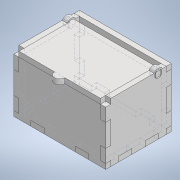
# Autodesk Inventor part: music box
Saved by Autodesk Inventor 2020 (Build 240168000, 168)
## iProperties
Created: 2021-07-07
Part Number: music box
Material: Generic
Document SubType Name: Modeling
Designer: Administrator
Density: 1 g/cm^3
Appearance: Default
Author: Administrator
Autodesk Inventor part; units mm, degrees
ref_plane "YZ Plane" through (0, 0, 0) normal (1, 0, 0) x (0, 1, 0)
ref_plane "XZ Plane" through (0, 0, 0) normal (0, 1, 0) x (-1, 0, 0)
ref_plane "XY Plane" through (0, 0, 0) normal (0, 0, 1) x (1, 0, 0)
sketch "Sketch1" plane through (0, 0, 0) normal (0, 0, 1) x (1, 0, 0)
  line L0 (-35, -22.5) -> (35, -22.5)
  line L1 (35, -22.5) -> (35, 22.5)
  line L2 (35, 22.5) -> (-35, 22.5)
  line L3 (-35, 22.5) -> (-35, -22.5)
  line L4 (-35, -22.5) -> (35, 22.5) construction
  line L5 (35, -22.5) -> (-35, 22.5) construction
  line L6 (-35, 0) -> (35, 0) construction
  line L7 (0, 22.5) -> (0, -22.5) construction
  line L8 (-35, 18.6) -> (-31.1, 18.6)
  line L9 (-31.1, 18.6) -> (-31.1, 8.6)
  line L10 (-31.1, 8.6) -> (-35, 8.6)
  line L11 (-35, 8.6) -> (-35, 18.6)
  line L12 (-35, -18.6) -> (-31.1, -18.6)
  line L13 (-31.1, -18.6) -> (-31.1, -8.6)
  line L14 (-31.1, -8.6) -> (-35, -8.6)
  line L15 (35, 18.6) -> (31.1, 18.6)
  line L16 (31.1, 18.6) -> (31.1, 8.6)
  line L17 (31.1, 8.6) -> (35, 8.6)
  line L18 (31.1, -18.6) -> (31.1, -8.6)
  line L19 (31.1, -8.6) -> (35, -8.6)
  line L20 (35, -18.6) -> (31.1, -18.6)
  line L21 (-22, -22.5) -> (-12, -22.5)
  line L22 (-12, -22.5) -> (-12, -18.6)
  line L23 (-12, -18.6) -> (-22, -18.6)
  line L24 (-22, -18.6) -> (-22, -22.5)
  line L25 (12, -22.5) -> (12, -18.6)
  line L26 (12, -18.6) -> (22, -18.6)
  line L27 (22, -18.6) -> (22, -22.5)
  point P0 (0, 0)
  point P1 (-35, -18.6)
  point P2 (35, -18.6)
  point P3 (35, -8.6)
  point P4 (35, 8.6)
  point P5 (35, 18.6)
  point P6 (-35, 8.6)
  point P7 (-35, -8.6)
  dimension "d0" = 70
  dimension "d1" = 45
  dimension "d2" = 3.9
  dimension "d3" = 10
  dimension "d4" = 3.9
  dimension "d7" = 10
  dimension "d8" = 3.9
  dimension "d9" = 12
  constraints: 56 end point, 16 symmetric about line, 6 midpoint, 6 parallel, 3 horizontal, 3 perpendicular, 2 point on line
  measures "d0" distance of L2.end L1.end
  measures "d1" distance of L1.end L0.end
  measures "d2" distance of L9.end L10.end
  measures "d3" distance of L8.end L9.end
  measures "d4" distance between parallel lines of L2 L8
  measures "d7" distance of L23.end L22.end
  measures "d8" distance of L22.end L21.end
  measures "d9" distance between parallel lines of L7 L22
extrude "Extrusion1" add sketch "Sketch1" along normal blind 3.9 contours L3 L12 L13 L14 L10 L9 L8 L2 L1 L15 L16 L17 L19 L18 L20 L0 L27 L26 L25 L22 L23 L24
sketch "Sketch2" plane through (-35, -8.6, 0) normal (-1, 0, 0) x (0, 0, 1)
  line L0 (50, -13.9) -> (0, -13.9)
  line L1 (0, -13.9) -> (0, 31.1)
  line L2 (0, 31.1) -> (50, 31.1)
  line L3 (50, 31.1) -> (50, -13.9)
  line L4 (50, -13.9) -> (0, 31.1) construction
  line L5 (0, -13.9) -> (50, 31.1) construction
  line L6 (3.9, 31.1) -> (3.9, 27.2) projected
  line L7 (0, 31.1) -> (0, 27.2) projected
  line L8 (3.9, 27.2) -> (0, 27.2)
  line L9 (0, 27.2) -> (0, 31.1)
  line L10 (0, 31.1) -> (3.9, 31.1)
  line L11 (3.9, 31.1) -> (3.9, 27.2)
  line L12 (25, 31.1) -> (25, -13.9) construction
  line L13 (0, 8.6) -> (50, 8.6) construction
  line L14 (0, 0) -> (0, -10) projected
  line L15 (0, -10) -> (3.9, -10)
  line L16 (3.9, -10) -> (3.9, -13.9)
  line L17 (3.9, -13.9) -> (0, -13.9)
  line L18 (0, -13.9) -> (0, -10)
  line L19 (0, 27.2) -> (0, 17.2) projected
  line L20 (3.9, 17.2) -> (3.9, 0) projected
  line L21 (0, 17.2) -> (3.9, 17.2)
  line L22 (3.9, 17.2) -> (3.9, 0)
  line L23 (3.9, 0) -> (0, 0)
  line L24 (0, 0) -> (0, 17.2)
  line L25 (46.1, 31.1) -> (46.1, 27.2)
  line L26 (46.1, 27.2) -> (50, 27.2)
  line L27 (50, -10) -> (46.1, -10)
  line L28 (46.1, -10) -> (46.1, -13.9)
  line L29 (46.1, 17.2) -> (46.1, 0)
  line L30 (50, 17.2) -> (46.1, 17.2)
  line L31 (46.1, 0) -> (50, 0)
  line L32 (10, -13.9) -> (20, -13.9)
  line L33 (20, -13.9) -> (20, -10)
  line L34 (20, -10) -> (10, -10)
  line L35 (10, -10) -> (10, -13.9)
  line L36 (50, 8.6) -> (0, 8.6) construction
  line L37 (30, -13.9) -> (30, -10)
  line L38 (30, -10) -> (40, -10)
  line L39 (40, -10) -> (40, -13.9)
  line L40 (7.9, 31.1) -> (11.8, 31.1)
  line L41 (11.8, 31.1) -> (11.8, 27.2) construction
  line L42 (11.8, 27.2) -> (7.9, 27.2) construction
  line L43 (7.9, 27.2) -> (7.9, 31.1) construction
  circle A0 centre (9.85, 29.15) radius 2.8
  circle A1 centre (9.85, 29.15) radius 3.8
  point P0 (25, 8.6)
  point P1 (0, 27.2)
  point P2 (20, -13.9)
  point P3 (30, -13.9)
  point P4 (6.5885, 31.1)
  point P5 (13.1115, 31.1)
  dimension "d10" = 50
  dimension "d11" = 45
  dimension "d12" = 10
  dimension "d13" = 3.9
  dimension "d14" = 5
  dimension "d28" = 3.9
  dimension "d29" = 3.9
  dimension "d30" = 4
  dimension "d31" = 5.6
  dimension "d32" = 1
  constraints: 78 end point, 17 symmetric about line, 12 parallel, 6 horizontal, 6 perpendicular, 5 midpoint, 2 centre point, 2 coincident, 2 point on line
  measures "d10" distance of L1.end L2.end
  measures "d11" distance of L2.end L0.start
  measures "d12" distance of L34.end L33.end
  measures "d13" distance of L33.end L32.end
  measures "d14" distance between parallel lines of L12 L33
  measures "d28" distance of L41.end L42.end
  measures "d29" distance of L40.end L41.end
  measures "d30" distance between parallel lines of L6 L43
  measures "d31" diameter of A0
  measures "d32" radial gap between concentric circles of A0 A1
extrude "Extrusion2" add sketch "Sketch2" against normal blind 3.9 separate body contours L0 L39 L38 L37 L33 L34 L35 L16 L15 L1 L23 L20 L21 L8 L6 L2 A1 L25 L26 L3 L30 L29 L31 L27 L28 | A1 L2 A0 | L2 A0 A1
mirror "Mirror1" about plane through (0, 0, 0) normal (1, 0, 0) of "Extrusion2" bodies 2
sketch "Sketch3" plane through (-35, 8.6, 50) normal (0, 0, 1) x (1, 0, 0)
  line L0 (0, 10) -> (3.9, 10) projected
  line L1 (57, -31.1) -> (70, -31.1) projected
  line L2 (0, 10) -> (70, 10)
  line L3 (70, 10) -> (70, -31.1)
  line L4 (70, -31.1) -> (0, -31.1)
  line L5 (0, -31.1) -> (0, 10)
  line L6 (0, 13.9) -> (0, 10) projected
  line L7 (3.9, 10) -> (3.9, 0) projected
  line L8 (0, 10) -> (3.9, 10)
  line L9 (3.9, 10) -> (3.9, 0)
  line L10 (3.9, 0) -> (0, 0)
  line L11 (0, 0) -> (0, 10)
  line L12 (0, 0) -> (0, -17.2) projected
  line L13 (3.9, -17.2) -> (3.9, -27.2) projected
  line L14 (0, -17.2) -> (3.9, -17.2)
  line L15 (3.9, -17.2) -> (3.9, -27.2)
  line L16 (3.9, -27.2) -> (0, -27.2)
  line L17 (0, -27.2) -> (0, -17.2)
  line L18 (66.1, 0) -> (66.1, 10) projected
  line L19 (70, 0) -> (70, 10) projected
  line L20 (66.1, 10) -> (70, 10)
  line L21 (70, 10) -> (70, 0)
  line L22 (70, 0) -> (66.1, 0)
  line L23 (66.1, 0) -> (66.1, 10)
  line L24 (66.1, -17.2) -> (66.1, 0) construction
  line L25 (66.1, -17.2) -> (70, -17.2)
  line L26 (70, -17.2) -> (70, -27.2)
  line L27 (70, -27.2) -> (66.1, -27.2)
  line L28 (66.1, -27.2) -> (66.1, -17.2)
  line L29 (13, -27.2) -> (23, -27.2) projected
  line L30 (13, -27.2) -> (23, -27.2)
  line L31 (23, -27.2) -> (23, -31.1)
  line L32 (23, -31.1) -> (13, -31.1)
  line L33 (13, -31.1) -> (13, -27.2)
  line L34 (47, -31.1) -> (47, -27.2) projected
  line L35 (57, -27.2) -> (57, -31.1) projected
  line L36 (47, -27.2) -> (57, -27.2)
  line L37 (57, -27.2) -> (57, -31.1)
  line L38 (57, -31.1) -> (47, -31.1)
  line L39 (47, -31.1) -> (47, -27.2)
  point P0 (35, -8.6)
  point P1 (0, 0)
  constraints: 56 end point, 14 parallel, 7 horizontal, 7 perpendicular, 2 point on line
extrude "Extrusion3" add sketch "Sketch3" against normal blind 3.9 separate body contours L2 L18 L22 L3 L25 L28 L27 L1 L35 L36 L34 L4 L31 L29 L33 L5 L16 L13 L14 L10 L7
sketch "Sketch4" plane through (-12, -22.5, 50) normal (0, -1, 0) x (1, 0, 0)
  line L0 (43.1, 0) -> (-19.1, 0) projected
  line L1 (12, 0) -> (12, -50) construction
  line L2 (47, -50) -> (-23, -50) construction
  line L3 (0, 0) -> (0, -3.9) projected
  line L4 (12, 0) -> (0, 0)
  line L5 (0, 0) -> (0, -3.9)
  line L6 (0, -3.9) -> (12, -3.9)
  line L7 (12, -3.9) -> (12, 0)
  line L8 (-10, 0) -> (-10, -3.9) projected
  line L9 (-23, 0) -> (-19.1, 0) projected
  line L10 (-10, -3.9) -> (-23, -3.9)
  line L11 (-23, -3.9) -> (-23, 0)
  line L12 (-23, 0) -> (-10, 0)
  line L13 (-10, 0) -> (-10, -3.9)
  line L14 (-23, -10) -> (-19.1, -10) projected
  line L15 (-19.1, -46.1) -> (-19.1, -3.9) projected
  line L16 (-23, -10) -> (-19.1, -10)
  line L17 (-19.1, -10) -> (-19.1, -3.9)
  line L18 (-19.1, -3.9) -> (-23, -3.9)
  line L19 (-23, -3.9) -> (-23, -10)
  line L20 (-23, -20) -> (-19.1, -20) projected
  line L21 (-23, -30) -> (-19.1, -30) projected
  line L22 (-23, -20) -> (-19.1, -20)
  line L23 (-19.1, -20) -> (-19.1, -30)
  line L24 (-19.1, -30) -> (-23, -30)
  line L25 (-23, -30) -> (-23, -20)
  line L26 (47, -46.1) -> (-23, -46.1) construction
  line L27 (12, -46.1) -> (0, -46.1)
  line L28 (0, -46.1) -> (0, -50)
  line L29 (0, -50) -> (12, -50)
  line L30 (12, -50) -> (12, -46.1)
  line L31 (-10, -50) -> (-10, -46.1) projected
  line L32 (-19.1, -50) -> (-23, -50) projected
  line L33 (-10, -46.1) -> (-23, -46.1)
  line L34 (-23, -46.1) -> (-23, -50)
  line L35 (-23, -50) -> (-10, -50)
  line L36 (-10, -50) -> (-10, -46.1)
  line L37 (-19.1, -50) -> (-19.1, -46.1) projected
  line L38 (-23, -40) -> (-19.1, -40) projected
  line L39 (-19.1, -46.1) -> (-23, -46.1)
  line L40 (-23, -46.1) -> (-23, -40)
  line L41 (-23, -40) -> (-19.1, -40)
  line L42 (-19.1, -40) -> (-19.1, -46.1)
  line L43 (34, 0) -> (34, -3.9)
  line L44 (34, -3.9) -> (47, -3.9)
  line L45 (47, -10) -> (43.1, -10)
  line L46 (43.1, -3.9) -> (47, -3.9)
  line L47 (47, -30) -> (43.1, -30)
  line L48 (47, -20) -> (43.1, -20)
  line L49 (34, -50) -> (34, -46.1)
  line L50 (43.1, -50) -> (43.1, -46.1)
  line L51 (47, -40) -> (43.1, -40)
  line L52 (24, 0) -> (24, -3.9)
  line L53 (12, 0) -> (24, 0)
  line L54 (24, -3.9) -> (12, -3.9)
  line L55 (43.1, -10) -> (43.1, -3.9)
  line L56 (43.1, -46.1) -> (43.1, -40)
  line L57 (43.1, -30) -> (43.1, -20)
  line L58 (34, -46.1) -> (47, -46.1)
  line L59 (34, -50) -> (47, -50)
  line L60 (-23, -46.1) -> (-10, -46.1)
  line L61 (0, -46.1) -> (12, -46.1)
  line L62 (-23, -50) -> (-10, -50)
  line L63 (0, -50) -> (12, -50)
  line L64 (-23, -50) -> (47, -50) construction
  line L65 (-23, -46.1) -> (47, -46.1) construction
  line L66 (12, -46.1) -> (24, -46.1)
  line L67 (24, -46.1) -> (24, -50)
  line L68 (24, -50) -> (12, -50)
  line L69 (-23, -3.9) -> (-23, 0) projected
  line L70 (47, -50) -> (47, -46.1) projected
  line L71 (-23, 0) -> (47, 0)
  line L72 (47, 0) -> (47, -50)
  line L73 (47, -50) -> (-23, -50)
  line L74 (-23, -50) -> (-23, 0)
  point P0 (47, -40)
  point P1 (47, -30)
  point P2 (47, -20)
  point P3 (47, -10)
  point P4 (34, 0)
  point P5 (24, 0)
  point P6 (-23, -20)
  point P7 (-23, -30)
  constraints: 118 end point, 30 symmetric about line, 16 parallel, 9 perpendicular, 8 horizontal, 3 point on line, 2 midpoint
extrude "Extrusion4" add sketch "Sketch4" against normal blind 3.9 separate body contours L43 L44 L55 L45 L72 L48 L57 L47 L51 L56 L58 L49 L73 L67 L66 L27 L28 L31 L33 L15 L10 L8 L0 L3 L6 L54 L52 | L15 L20 L74 L14 | L15 L38 L74 L21
sketch "Sketch5" plane through (-31.1, 18.6, 50) normal (0, 1, 0) x (1, 0, 0)
  line L0 (-3.9, 0) -> (0, 0) projected
  line L1 (62.2, 40) -> (62.2, 46.1) projected
  line L2 (62.2, 0) -> (62.2, 42.1)
  line L3 (62.2, 42.1) -> (0, 42.1)
  line L4 (0, 42.1) -> (0, 0)
  line L5 (66.1, 46.1) -> (-3.9, 46.1) projected
  line L6 (62.2, 0) -> (0, 0) projected
  arc A0 (27.2, 0) -> (35, 0) centre (31.1, 0) ccw
  line L7 (0, 0) -> (27.2, 0)
  line L8 (35, 0) -> (62.2, 0)
  line L9 (0, 42.1) -> (-3.9, 42.1)
  line L10 (-3.9, 42.1) -> (-3.9, 38.2)
  line L11 (-3.9, 38.2) -> (0, 38.2)
  line L12 (0, 38.2) -> (0, 42.1)
  line L13 (62.2, 42.1) -> (66.1, 42.1)
  line L14 (66.1, 42.1) -> (66.1, 38.2)
  line L15 (66.1, 38.2) -> (62.2, 38.2)
  line L16 (62.2, 38.2) -> (62.2, 42.1)
  point P0 (31.1, 50)
  point P1 (35, 0)
  point P2 (62.2, 38.2)
  point P3 (0, 38.2)
  dimension "d21" = 4
  dimension "d22" = 7.8
  dimension "d33" = 3.9
  dimension "d34" = 3.9
  dimension "d35" = 3.9
  dimension "d36" = 3.9
  constraints: 26 end point, 7 parallel, 4 horizontal, 4 perpendicular, 2 point on circle, 1 centre point, 1 midpoint, 1 point on line
  measures "d21" distance between parallel lines of L5 L3
  measures "d22" diameter of A0
  measures "d33" distance of L11.end L10.end
  measures "d34" distance of L10.end L9.end
  measures "d35" distance of L14.end L15.end
  measures "d36" distance of L13.end L14.end
extrude "Extrusion5" add sketch "Sketch5" along normal blind 3.9 separate body
equation "\"d0\" = length"
equation "\"d1\" = height"
equation "\"d2\" = thick"
equation "\"d3\" = tab"
equation "\"d4\" = thick"
equation "\"d7\" = tab"
equation "\"d8\" = thick"
equation "\"d5\" = thick"
equation "\"d10\" = witdh"
equation "\"d11\" = height"
equation "\"d12\" = tab"
equation "\"d13\" = thick"
equation "\"d28\" = thick"
equation "\"d29\" = thick"
equation "\"d15\" = thick"
equation "\"d17\" = thick"
equation "\"d19\" = thick"
equation "\"d33\" = thick"
equation "\"d34\" = thick"
equation "\"d35\" = thick"
equation "\"d36\" = thick"
equation "\"d23\" = thick"
equation "\"length\" = 70"
equation "\"witdh\" = 50"
equation "\"height\" = 45"
equation "\"thick\" = 3.9"
equation "\"tab\" = 10"
body "Solid1"
body "Solid2"
body "Solid3"
body "Solid4"
body "Solid5"
